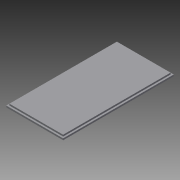
# Autodesk Inventor part: SD_BaseStation_Lid
Saved by Autodesk Inventor 2015 (Build 190159000, 159)
## iProperties
Created: 2014-04-30
Part Number: SD_BaseStation_Lid
Material: Generic
Document SubType Name: Modeling
Designer: xbmc
Density: 1 g/cm^3
Appearance: Default
Author: xbmc
Autodesk Inventor part; units mm, degrees
ref_plane "YZ Plane" through (0, 0, 0) normal (1, 0, 0) x (0, 1, 0)
ref_plane "XZ Plane" through (0, 0, 0) normal (0, 1, 0) x (-1, 0, 0)
ref_plane "XY Plane" through (0, 0, 0) normal (0, 0, 1) x (1, 0, 0)
sketch "Sketch1" plane through (0, 0, 0) normal (0, 1, 0) x (-1, 0, 0)
  line L0 (33.1574, 54.0426) -> (-23.9926, 54.0426)
  line L1 (-23.9926, 54.0426) -> (-23.9926, -57.0824)
  line L2 (-23.9926, -57.0824) -> (33.1574, -57.0824)
  line L3 (33.1574, -57.0824) -> (33.1574, 54.0426)
  point P0 (0, 0)
  dimension "d0" = 111.125
  dimension "d1" = 57.15
  constraints: 8 end point, 2 parallel, 1 horizontal, 1 perpendicular
  measures "d0" distance of L2.end L0.start
  measures "d1" distance of L1.end L2.end
extrude "Extrusion1" add sketch "Sketch1" along normal blind 1.5875
sketch "Sketch2" plane through (0, 1.5875, 0) normal (0, 1, 0) x (1, 0, 0)
  line L0 (-31.5699, -52.4551) -> (22.4051, -52.4551)
  line L1 (22.4051, -52.4551) -> (22.4051, 55.4949)
  line L2 (22.4051, 55.4949) -> (-31.5699, 55.4949)
  line L3 (-31.5699, 55.4949) -> (-31.5699, -52.4551)
  line L4 (-33.1574, -54.0426) -> (23.9926, -54.0426) projected
  line L5 (23.9926, -54.0426) -> (23.9926, 57.0824) projected
  line L6 (23.9926, 57.0824) -> (-33.1574, 57.0824) projected
  line L7 (-33.1574, 57.0824) -> (-33.1574, -54.0426) projected
  point P0 (0, 0)
  dimension "d4" = 1.5875
  dimension "d5" = 1.5875
  dimension "d6" = 1.5875
  dimension "d7" = 1.5875
  constraints: 8 end point, 2 parallel, 1 horizontal, 1 perpendicular
  measures "d4" distance between parallel lines of L4 L0
  measures "d5" distance between parallel lines of L5 L1
  measures "d6" distance between parallel lines of L6 L2
  measures "d7" distance between parallel lines of L7 L3
extrude "Extrusion2" add sketch "Sketch2" along normal blind 1.5875 contours L3 L2 L1 L0
body "Solid1"
